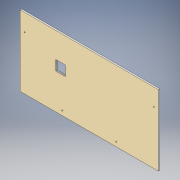
# Autodesk Inventor part: Half Ceiling Model 2
Saved by Autodesk Inventor 2017 (Build 210142000, 142)
## iProperties
Created: 2017-05-30
Part Number: Half Ceiling Model 2
Material: Generic
Document SubType Name: Modeling
Designer: cas7
Density: 1 g/cm^3
Appearance: Default
Mass: 15843 g
Surface Area: 20630 cm^2
Volume: 15843 cm^3
Author: cas7
Autodesk Inventor part; units mm, degrees
ref_plane "YZ Plane" through (0, 0, 0) normal (1, 0, 0) x (0, 1, 0)
ref_plane "XZ Plane" through (0, 0, 0) normal (0, 1, 0) x (-1, 0, 0)
ref_plane "XY Plane" through (0, 0, 0) normal (0, 0, 1) x (1, 0, 0)
sketch "Sketch1" plane through (0, 0, 0) normal (0, 0, 1) x (1, 0, 0)
  line L0 (0, 0) -> (1397, 0)
  line L1 (1397, 0) -> (1397, 714.375)
  line L2 (1397, 714.375) -> (0, 714.375)
  line L3 (0, 714.375) -> (0, 0)
  dimension "d0" = 1397
  dimension "d1" = 714.375
  constraints: 8 end point, 2 parallel, 1 horizontal, 1 perpendicular
  measures "d0" distance of L2.end L1.end
  measures "d1" distance of L1.end L0.end
extrude "Extrusion1" add sketch "Sketch1" along normal blind 15.875
sketch "Sketch10" plane through (0, 0, 15.875) normal (0, 0, 1) x (1, 0, 0)
  line L0 (0, 0) -> (1397, 0) projected
  line L1 (1397, 0) -> (1397, 714.375) projected
  line L2 (0, 714.375) -> (0, 0) projected
  line L3 (0, 540.5628) -> (44.45, 540.5628)
  line L4 (425.45, 0) -> (425.45, 44.45)
  line L5 (971.55, 0) -> (971.55, 44.45)
  line L6 (1397, 540.5628) -> (1352.55, 540.5628)
  dimension "d68" = 44.45
  dimension "d69" = 44.45
  dimension "d70" = 44.45
  dimension "d71" = 44.45
  constraints: 8 end point, 4 coincident, 4 point on line, 2 perpendicular, 1 horizontal, 1 vertical
  measures "d68" distance of L3.start L3.end
  measures "d69" distance of L4.start L4.end
  measures "d70" distance of L5.start L5.end
  measures "d71" distance of L6.start L6.end
hole "Hole4" at (44.45, 540.5628, 15.875) at (425.45, 44.45, 15.875) at (971.55, 44.45, 15.875) at (1352.55, 540.5628, 15.875) direction (0, 0, -1) diameter 10.5918 depth 35.179 tip angle 118 thread size "1/2-13 UNC" class "2B" standard "ANSI Unified Screw Threads"
sketch "Sketch15" plane through (0, 0, 15.875) normal (0, 0, 1) x (1, 0, 0)
  line L0 (0, 714.375) -> (0, 0) projected
  line L1 (0, 0) -> (88.9, 0)
  line L2 (0, 0) -> (1397, 0) projected
  line L3 (88.9, 0) -> (104.775, 0)
  line L4 (104.775, 0) -> (409.575, 0)
  line L5 (409.575, 0) -> (409.575, 409.575)
  line L6 (359.575, 359.575) -> (459.575, 359.575)
  line L7 (459.575, 359.575) -> (459.575, 459.575)
  line L8 (459.575, 459.575) -> (359.575, 459.575)
  line L9 (359.575, 459.575) -> (359.575, 359.575)
  line L10 (359.575, 359.575) -> (459.575, 459.575) construction
  line L11 (459.575, 359.575) -> (359.575, 459.575) construction
  dimension "d107" = 88.9
  dimension "d108" = 15.875
  dimension "d109" = 304.8
  dimension "d110" = 409.575
  dimension "d111" = 100
  dimension "d112" = 100
  constraints: 20 end point, 3 point on line, 2 midpoint, 2 parallel, 2 perpendicular, 1 horizontal
  measures "d107" distance of L0.end L1.end
  measures "d108" distance of L1.end L3.end
  measures "d109" distance of L3.end L4.end
  measures "d110" distance of L4.end L5.end
  measures "d111" distance of L8.end L7.end
  measures "d112" distance of L7.end L6.end
extrude "Extrusion6" cut sketch "Sketch15" against normal blind 15.875
body "Solid1"
